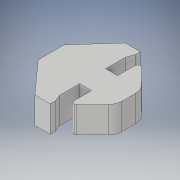
# Autodesk Inventor part: sliding_t_nut_prototype01
Saved by Autodesk Inventor 2017 (Build 210142000, 142)
## iProperties
Created: 2016-08-18
Part Number: sliding_t_nut_prototype01
Material: Generic
Document SubType Name: Modeling
Designer: jvoigts
Density: 1 g/cm^3
Appearance: Default
Author: jvoigts
Autodesk Inventor part; units mm, degrees
ref_plane "YZ Plane" through (0, 0, 0) normal (1, 0, 0) x (0, 1, 0)
ref_plane "XZ Plane" through (0, 0, 0) normal (0, 1, 0) x (-1, 0, 0)
ref_plane "XY Plane" through (0, 0, 0) normal (0, 0, 1) x (1, 0, 0)
sketch "Sketch1" plane through (0, 0, 0) normal (0, 1, 0) x (-1, 0, 0)
  line L0 (-12.7, 12.7) -> (12.7, 12.7)
  line L1 (12.7, 12.7) -> (12.7, -12.7)
  line L2 (12.7, -12.7) -> (-12.7, -12.7)
  line L3 (-12.7, -12.7) -> (-12.7, 12.7)
  line L4 (-12.7, 12.7) -> (12.7, -12.7) construction
  line L5 (12.7, 12.7) -> (-12.7, -12.7) construction
  line L6 (14.9209, 3.2512) -> (10.4791, 3.2512)
  line L7 (10.4791, 3.2512) -> (10.4791, -3.2512)
  line L8 (10.4791, -3.2512) -> (14.9209, -3.2512)
  line L9 (14.9209, -3.2512) -> (14.9209, 3.2512)
  line L10 (14.9209, 3.2512) -> (10.4791, -3.2512) construction
  line L11 (10.4791, 3.2512) -> (14.9209, -3.2512) construction
  line L12 (12.7, 3.2512) -> (10.4902, 3.2512)
  line L13 (10.4902, 3.2512) -> (10.4902, 9.3687)
  line L14 (10.4902, 9.3687) -> (12.7, 9.3687)
  line L15 (12.7, 9.3687) -> (12.7, 3.2512)
  line L16 (-4.5426, 4.5426) -> (4.5426, 4.5426)
  line L17 (4.5426, 1.686) -> (4.5426, -1.686)
  line L18 (4.5426, -4.5426) -> (-4.5426, -4.5426)
  line L19 (-4.5426, -4.5426) -> (-4.5426, 4.5426)
  line L20 (-4.5426, 4.5426) -> (4.5426, -4.5426) construction
  line L21 (4.5426, 4.5426) -> (-4.5426, -4.5426) construction
  line L22 (12.7, 12.7) -> (-12.7, -12.7) construction
  line L23 (11.9293, 13.4707) -> (-13.4707, -11.9293)
  line L24 (5.4725, 3.9311) -> (13.4707, 11.9293)
  arc A0 (13.4707, 11.9293) -> (11.9293, 13.4707) centre (12.7, 12.7) ccw
  arc A1 (-13.4707, -11.9293) -> (-11.9293, -13.4707) centre (-12.7, -12.7) ccw
  line L25 (12.7, -12.7) -> (-12.7, 12.7) construction
  line L26 (11.9293, -13.4707) -> (-13.4707, 11.9293)
  line L27 (5.4725, -3.9311) -> (13.4707, -11.9293)
  arc A2 (11.9293, -13.4707) -> (13.4707, -11.9293) centre (12.7, -12.7) ccw
  arc A3 (-11.9293, 13.4707) -> (-13.4707, 11.9293) centre (-12.7, 12.7) ccw
  arc A4 (5.4725, 3.9311) -> (4.5426, 1.686) centre (7.7176, 1.686) ccw
  arc A5 (4.5426, -1.686) -> (5.4725, -3.9311) centre (7.7176, -1.686) ccw
  point P0 (0, 0)
  point P1 (12.7, 0)
  point P2 (0, 0)
  point P3 (0, 0)
  dimension "d0" = 25.4
  dimension "d1" = 25.4
  dimension "d2" = 6.5024
  dimension "d3" = 2.2098
  dimension "d4" = 3.175
  constraints: 60 end point, 12 point on circle, 12 tangent, 10 midpoint, 10 parallel, 6 centre point, 5 point on line, 4 horizontal, 4 perpendicular, 2 collinear, 1 equal radius
  measures "d0" distance of L0.end L1.end
  measures "d1" distance of L1.end L2.end
  measures "d2" distance of L8.end L6.start
  measures "d3" distance of L13.end L14.end
  measures "d4" radius of A4
sketch "Sketch2" plane through (0, 0, 0) normal (0, 1, 0) x (-1, 0, 0)
  line L0 (9.3228, 7.7741) -> (5.6047, 4.0154)
  line L1 (5.6047, 4.0154) -> (5.5129, 3.9226)
  line L2 (4.5951, 1.6897) -> (4.5951, 0)
  line L3 (9.7743, 7.9625) -> (9.7971, 7.9625)
  line L4 (10.4321, 7.3275) -> (10.4321, 3.1448)
  line L5 (10.4321, 3.1448) -> (13.3143, 3.1448)
  arc A0 (5.5129, 3.9226) -> (4.5951, 1.6897) centre (7.7701, 1.6897) ccw
  arc A1 (9.7743, 7.9625) -> (9.3228, 7.7741) centre (9.7743, 7.3275) ccw
  arc A2 (10.4321, 7.3275) -> (9.7971, 7.9625) centre (9.7971, 7.3275) ccw
  line L6 (13.3143, 3.1448) -> (13.3143, 7.9625)
  line L7 (13.3143, 7.9625) -> (12.6666, 9.6561)
  line L8 (12.6666, 9.6561) -> (12.6666, 10.8508)
  line L9 (12.6666, 10.8508) -> (14.9475, 10.8508)
  line L10 (14.9475, 10.8508) -> (16.328, 10.8508)
  line L11 (16.328, 10.8508) -> (23.2713, 3.1448)
  line L12 (23.2713, 3.1448) -> (23.2713, 0)
  line L13 (9.3228, -7.7741) -> (5.6047, -4.0154)
  line L14 (4.5951, -1.6897) -> (4.5951, 0)
  line L15 (10.4321, -7.3275) -> (10.4321, -3.1448)
  line L16 (10.4321, -3.1448) -> (13.3143, -3.1448)
  arc A3 (4.5951, -1.6897) -> (5.5129, -3.9226) centre (7.7701, -1.6897) ccw
  arc A4 (9.3228, -7.7741) -> (9.7743, -7.9625) centre (9.7743, -7.3275) ccw
  arc A5 (9.7971, -7.9625) -> (10.4321, -7.3275) centre (9.7971, -7.3275) ccw
  line L17 (13.3143, -3.1448) -> (13.3143, -7.9625)
  line L18 (13.3143, -7.9625) -> (12.6666, -9.6561)
  line L19 (12.6666, -9.6561) -> (12.6666, -10.8508)
  line L20 (12.6666, -10.8508) -> (14.9475, -10.8508)
  line L21 (14.9475, -10.8508) -> (16.328, -10.8508)
  line L22 (16.328, -10.8508) -> (23.2713, -3.1448)
  line L23 (23.2713, -3.1448) -> (23.2713, 0)
  line L24 (5.5129, -3.9226) -> (5.6047, -4.0154)
  line L25 (9.7971, -7.9625) -> (9.7743, -7.9625)
  point P0 (0, 0)
  point P1 (4.5951, 2.9948)
  dimension "d5" = 3.175
  dimension "d6" = 0.635
  constraints: 52 end point, 12 point on circle, 6 centre point, 6 tangent, 5 point on line, 3 perpendicular, 3 vertical, 2 horizontal, 1 equal radius, 1 parallel
  measures "d5" radius of A0
  measures "d6" radius of A1
extrude "Extrusion1" add sketch "Sketch2" along normal blind 6.35
body "Solid1"
